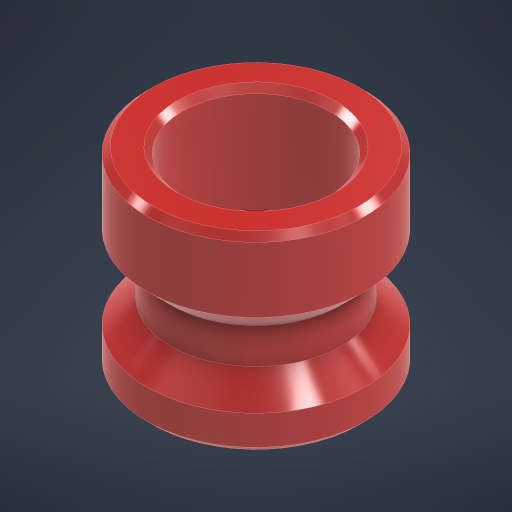
# Autodesk Inventor part: Z25_Side_Lock_Button
Saved by Autodesk Inventor 2025 (Build 290162010, 162A)
## iProperties
Created: 2023-02-13
Part Number: Z25_Side_Lock_Button
Material: Aluminum 6061
Document SubType Name: Modeling
Designer: dzw04
Density: 2.7 g/cm^3
Appearance: Orange-Red
Author: dzw04
Autodesk Inventor part; units mm, degrees
ref_plane "YZ Plane" through (0, 0, 0) normal (1, 0, 0) x (0, 1, 0)
ref_plane "XZ Plane" through (0, 0, 0) normal (0, 1, 0) x (-1, 0, 0)
ref_plane "XY Plane" through (0, 0, 0) normal (0, 0, 1) x (1, 0, 0)
sketch "Sketch1" plane through (0, 0, 0) normal (0, 0, 1) x (1, 0, 0)
  line L0 (0, 0) -> (-1.6, 0) construction
  line L1 (0, 0) -> (0, 8)
  line L2 (-1.6, 0) -> (-4.6, 0)
  line L3 (-1.6, 0) -> (-1.6, 3.5)
  line L4 (-1.6, 3.5) -> (-3.1, 3.5)
  line L5 (-3.1, 3.5) -> (-3.1, 8)
  line L6 (-3.1, 8) -> (-4.6, 8)
  line L7 (-4.6, 8) -> (-4.6, 4)
  line L8 (-4.6, 4) -> (-3.6, 4)
  line L9 (-3.6, 4) -> (-3.6, 2.5)
  line L10 (-3.6, 2.5) -> (-4.6, 2.5)
  line L11 (-4.6, 2.5) -> (-4.6, 0)
  dimension "d0" = 1.6
  dimension "d1" = 8
  dimension "d2" = 3
  dimension "d3" = 3.5
  dimension "d4" = 1.5
  dimension "d5" = 4
  dimension "d6" = 1
  dimension "d7" = 1.5
  constraints: 24 end point, 6 perpendicular, 2 horizontal, 2 parallel, 2 vertical, 1 point on line
  measures "d0" distance of L0.start L0.end
  measures "d1" distance of L0.start L1.end
  measures "d2" distance of L0.end L2.end
  measures "d3" distance of L0.end L3.end
  measures "d4" distance of L3.end L4.end
  measures "d5" distance of L6.end L7.end
  measures "d6" distance of L7.end L8.end
  measures "d7" distance of L8.end L9.end
revolve "Revolution1" add sketch "Sketch1" angle 360 about axis through (0, 0, 0) along (0, 1, 0)
chamfer "Chamfer1" distance 1 angle 45 2 edges at (4.6, 2.5, 0) (4.6, 4, 0)
chamfer "Chamfer2" distance 0.25 angle 45 4 edges at (4.6, 8, 0) (3.1, 8, 0) (4.6, 0, 0) (1.6, 0, 0)
body "Solid1"
